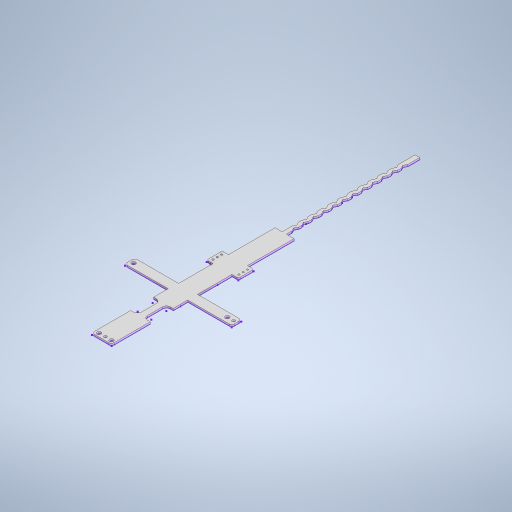
# Autodesk Inventor part: Thumb Finger Part
Saved by Autodesk Inventor 2023.1 (Build 271208000, 208)
## iProperties
Created: 2022-09-21
Part Number: Thumb Finger Part
Material: Generic
Document SubType Name: Modeling
Designer: lxpe222
Density: 1 g/cm^3
Appearance: Default
Author: lxpe222
Autodesk Inventor part; units mm, degrees
ref_plane "YZ Plane" through (0, 0, 0) normal (1, 0, 0) x (0, 1, 0)
ref_plane "XZ Plane" through (0, 0, 0) normal (0, 1, 0) x (-1, 0, 0)
ref_plane "XY Plane" through (0, 0, 0) normal (0, 0, 1) x (1, 0, 0)
sketch "Sketch1" plane through (0, 0, 0) normal (0, 1, 0) x (-1, 0, 0)
  line L0 (-8.7606, 60.7366) -> (-8.7606, 52.244)
  line L1 (2.2646, -7.3452) -> (2.2646, 17.544)
  line L2 (-8.811, 74.1038) -> (-8.811, 95.1313)
  line L3 (-7.311, 96.6313) -> (1.089, 96.6313)
  line L4 (2.589, 95.1313) -> (2.589, 74.061)
  circle A0 centre (0.414, 94.6613) radius 1.175
  circle A1 centre (-6.816, 94.6613) radius 1.175
  line L5 (-8.7606, 60.7366) -> (-7.0943, 60.7366)
  line L6 (-4.8143, 63.0166) -> (-4.8143, 71.8238)
  line L7 (-7.0943, 74.1038) -> (-8.811, 74.1038)
  line L8 (2.589, 74.061) -> (0.9294, 74.061)
  line L9 (-1.3506, 71.781) -> (-1.3506, 63.0166)
  line L10 (0.9294, 60.7366) -> (2.6222, 60.7366)
  arc A2 (0.9294, 74.061) -> (-1.3506, 71.781) centre (0.9294, 71.781) ccw
  arc A3 (-1.3506, 63.0166) -> (0.9294, 60.7366) centre (0.9294, 63.0166) ccw
  arc A4 (-7.0943, 60.7366) -> (-4.8143, 63.0166) centre (-7.0943, 63.0166) ccw
  arc A5 (-4.8143, 71.8238) -> (-7.0943, 74.1038) centre (-7.0943, 71.8238) ccw
  line L11 (2.6222, 52.244) -> (26.2646, 52.244)
  line L12 (27.7646, 50.744) -> (27.7646, 48.044)
  line L13 (26.2646, 46.544) -> (2.2646, 46.544)
  line L14 (-8.7606, 52.244) -> (-32.7606, 52.244)
  line L15 (-34.2606, 50.744) -> (-34.2606, 48.044)
  line L16 (-32.7606, 46.544) -> (-8.7606, 46.544)
  line L17 (2.2646, 26.544) -> (4.9546, 26.544)
  line L18 (5.9546, 25.544) -> (5.9546, 18.544)
  line L19 (4.9546, 17.544) -> (2.2646, 17.544)
  line L20 (-8.7606, 26.544) -> (-11.4506, 26.544)
  line L21 (-12.4506, 25.544) -> (-12.4506, 18.544)
  line L22 (-11.4506, 17.544) -> (-8.7606, 17.544)
  circle A6 centre (-3.2163, 94.6113) radius 0.85
  circle A7 centre (-28.8843, 49.394) radius 1.2
  circle A8 centre (-32.5093, 49.394) radius 0.825
  circle A9 centre (25.5896, 49.394) radius 1.2
  line L23 (2.6222, 52.244) -> (2.6222, 60.7366)
  line L24 (-8.7606, 17.544) -> (-8.7606, -9.5531)
  arc A10 (2.589, 95.1313) -> (1.089, 96.6313) centre (1.089, 95.1313) ccw
  arc A11 (-7.311, 96.6313) -> (-8.811, 95.1313) centre (-7.311, 95.1313) ccw
  arc A12 (26.2646, 46.544) -> (27.7646, 48.044) centre (26.2646, 48.044) ccw
  arc A13 (27.7646, 50.744) -> (26.2646, 52.244) centre (26.2646, 50.744) ccw
  arc A14 (-34.2606, 48.044) -> (-32.7606, 46.544) centre (-32.7606, 48.044) ccw
  arc A15 (-32.7606, 52.244) -> (-34.2606, 50.744) centre (-32.7606, 50.744) ccw
  line L25 (-4.2606, -9.5527) -> (-4.2468, -12.4286)
  line L26 (-1.8233, -14.9375) -> (-1.8491, -9.5528)
  line L27 (-8.7606, -9.5531) -> (-4.2606, -9.5528)
  line L28 (-4.2167, -68.4873) -> (-4.2167, -70.4904)
  line L29 (-2.7339, -69.436) -> (-1.6273, -67.5846)
  line L30 (-3.1633, -66.6169) -> (-4.2167, -68.4873)
  line L31 (-1.6273, -65.5835) -> (-1.6273, -67.5846)
  line L32 (-3.1633, -66.6169) -> (-4.2167, -64.7373)
  line L33 (-2.6377, -63.8108) -> (-1.6273, -65.5835)
  line L34 (-4.2167, -64.7373) -> (-4.2167, -62.7373)
  line L35 (-1.701, -26.8084) -> (-2.7095, -28.7084)
  line L36 (-4.2214, -28.1115) -> (-4.2214, -30.1115)
  line L37 (-2.7095, -28.7084) -> (-1.6807, -30.5584)
  line L38 (-1.6807, -32.5584) -> (-1.6807, -30.5584)
  line L39 (-3.1648, -32.0115) -> (-4.2214, -30.1115)
  line L40 (-1.6896, -38.3084) -> (-2.7534, -40.2084)
  line L41 (-2.7534, -40.2084) -> (-1.6666, -42.0584)
  line L42 (-3.1482, -43.5109) -> (-4.2333, -41.6115)
  line L43 (-1.6666, -44.0584) -> (-1.6666, -42.0584)
  line L44 (-1.6666, -44.0584) -> (-2.7357, -45.9584)
  line L45 (-4.299, -45.3609) -> (-3.1482, -43.5109)
  line L46 (-4.2333, -39.6115) -> (-4.2333, -41.6115)
  line L47 (-4.2333, -39.6115) -> (-3.1706, -37.7615)
  line L48 (-1.6896, -38.3084) -> (-1.6896, -36.3084)
  line L49 (-3.1706, -37.7615) -> (-4.2244, -35.8615)
  line L50 (-2.7156, -34.4584) -> (-1.6896, -36.3084)
  line L51 (-4.2244, -33.8615) -> (-4.2244, -35.8615)
  line L52 (-3.2118, -14.7615) -> (-0.6911, -14.7642) construction
  line L53 (-4.2824, -16.6115) -> (-3.2118, -14.7615)
  line L54 (-4.2824, -16.6115) -> (-4.2824, -18.6115)
  line L55 (-2.8081, -17.2084) -> (-1.731, -19.0584)
  line L56 (-3.2222, -20.5115) -> (-4.2824, -18.6115)
  line L57 (-1.731, -21.0584) -> (-1.731, -19.0584)
  line L58 (-3.2118, -14.7615) -> (-4.2468, -12.9643)
  line L59 (-4.2214, -28.1115) -> (-3.1802, -26.2615)
  line L60 (-1.701, -26.8084) -> (-1.701, -24.8084)
  line L61 (-3.1802, -26.2615) -> (-4.2412, -24.3615)
  line L62 (-2.7341, -22.9584) -> (-1.701, -24.8084)
  line L63 (-4.2412, -22.3615) -> (-4.2412, -24.3615)
  line L64 (-4.2412, -22.3615) -> (-3.2222, -20.5115)
  line L65 (-1.731, -21.0584) -> (-2.7341, -22.9584)
  line L66 (-3.1743, -49.2607) -> (-4.299, -47.3609)
  line L67 (-4.3381, -51.1107) -> (-3.1743, -49.2607)
  line L68 (-2.6912, -52.2338) -> (-1.5867, -54.0838)
  line L69 (-4.3381, -51.1107) -> (-4.3381, -53.1107)
  line L70 (-1.7329, -50.3338) -> (-2.6912, -52.2338)
  line L71 (-1.7329, -50.3338) -> (-1.6601, -49.8084)
  line L72 (-1.6601, -49.8084) -> (-1.6601, -47.8084)
  line L73 (-2.7357, -45.9584) -> (-1.6601, -47.8084)
  line L74 (-4.299, -45.3609) -> (-4.299, -47.3609)
  line L75 (-1.6807, -32.5584) -> (-2.7156, -34.4584)
  line L76 (-4.2244, -33.8615) -> (-3.1648, -32.0115)
  line L77 (-2.7339, -69.436) -> (-1.7343, -71.333)
  line L78 (-3.2659, -72.3279) -> (-4.2167, -70.4904)
  line L79 (-1.7343, -71.333) -> (-1.7343, -73.333)
  line L80 (-3.2659, -72.3279) -> (-4.425, -74.2346)
  line L81 (-2.7876, -75.2268) -> (-1.7343, -73.333)
  line L82 (-2.7876, -75.2268) -> (-1.7343, -77.083)
  line L83 (-4.425, -74.2346) -> (-4.425, -76.2346)
  line L84 (-3.2287, -55.1137) -> (-4.3381, -53.1107)
  line L85 (-1.5867, -54.0838) -> (-1.5867, -56.0838)
  line L86 (-3.2287, -55.1137) -> (-4.3098, -56.9885)
  line L87 (-2.6396, -58.004) -> (-1.5867, -56.0838)
  line L88 (-4.3098, -56.9885) -> (-4.313, -58.9885)
  line L89 (-2.6396, -58.004) -> (-1.5867, -59.8338)
  line L90 (-3.2112, -60.8694) -> (-4.313, -58.9885)
  line L91 (-3.2112, -60.8694) -> (-4.2167, -62.7373)
  line L92 (-2.6377, -63.8108) -> (-1.5867, -61.8338)
  line L93 (-1.5867, -59.8338) -> (-1.5867, -61.8338)
  line L94 (-3.372, -78.0699) -> (-4.425, -79.9846)
  line L95 (-3.372, -78.0699) -> (-4.425, -76.2346)
  line L96 (-4.425, -86.9746) -> (-4.425, -79.9846)
  line L97 (-1.7343, -86.9746) -> (-4.425, -86.9746)
  line L98 (-1.7343, -77.083) -> (-1.7343, -86.9746)
  line L99 (-1.8233, -14.9375) -> (-1.8233, -15.4921)
  line L100 (-1.8233, -15.4921) -> (-2.8081, -17.2084)
  line L101 (-4.2468, -12.4286) -> (-4.2468, -12.9643)
  line L102 (-1.8491, -9.5528) -> (2.2646, -9.5528)
  line L103 (2.2646, -9.5528) -> (2.2646, -7.3452)
  line L104 (2.2646, 26.544) -> (2.2646, 46.544)
  line L105 (-8.7606, 26.544) -> (-8.7606, 46.544)
  circle A16 centre (4.2946, 22.044) radius 0.5
  circle A17 centre (4.2946, 19.544) radius 0.5
  circle A18 centre (4.2946, 24.544) radius 0.5
  circle A19 centre (-10.7906, 22.044) radius 0.5
  circle A20 centre (-10.7906, 19.544) radius 0.5
  circle A21 centre (-10.7906, 24.544) radius 0.5
  arc A22 (4.9546, 17.544) -> (5.9546, 18.544) centre (4.9546, 18.544) ccw
  arc A23 (5.9546, 25.544) -> (4.9546, 26.544) centre (4.9546, 25.544) ccw
  arc A24 (-11.4506, 26.544) -> (-12.4506, 25.544) centre (-11.4506, 25.544) ccw
  arc A25 (-12.4506, 18.544) -> (-11.4506, 17.544) centre (-11.4506, 18.544) ccw
  point P0 (-8.811, 96.6313)
  point P1 (2.589, 96.6313)
  point P2 (-6.9279, 18.3671)
  point P3 (0.6606, 18.3671)
  point P4 (-6.9323, 25.0551)
  point P5 (27.7646, 46.544)
  point P6 (27.7646, 52.244)
  point P7 (-34.2606, 46.544)
  point P8 (-34.2606, 52.244)
  point P9 (2.2646, 46.9721)
  point P10 (-8.7606, 35.0882)
  point P11 (5.9546, 17.544)
  point P12 (5.9546, 26.544)
  point P13 (-12.4506, 17.544)
  point P14 (-12.4506, 26.544)
  point P15 (-3.6908, -42.5612)
  point P16 (-3.7523, -19.5615)
  point P17 (-3.7317, -21.4365)
  point P18 (-3.7367, -48.3108)
  point P19 (-2.139, -53.1588)
  point P20 (2.6394, 52.7)
  point P21 (-8.7606, 56.4903)
  point P22 (3.6096, 26.544)
  dimension "d276" = 2.4
  dimension "d277" = 2.4
  dimension "d280" = 1.5
  dimension "d281" = 2.35
  dimension "d282" = 2.35
  dimension "d284" = 1.65
  dimension "d286" = 1.7
  dimension "d288" = 0.795
  dimension "d289" = 0.795
  dimension "d290" = 1.17
  dimension "d291" = 1.6
  dimension "d292" = 1.575
  dimension "d293" = 1.5
  dimension "d294" = 1.5
  dimension "d296" = 0.975
  dimension "d297" = 2.175
  dimension "d312" = 0.9263
  dimension "d313" = 120
  dimension "d315" = 2
  dimension "d316" = 2
  dimension "d317" = 2
  dimension "d318" = 2
  dimension "d319" = 2
  dimension "d320" = 2
  dimension "d321" = 2
  dimension "d322" = 2
  dimension "d323" = 2
  dimension "d324" = 2
  dimension "d325" = 2
  dimension "d326" = 2
  dimension "d327" = 2
  dimension "d328" = 2
  dimension "d329" = 2
  dimension "d330" = 2.0032
  dimension "d331" = 2
  dimension "d332" = 2
  dimension "d333" = 3.75
  dimension "d334" = 3.75
  dimension "d335" = 3.75
  dimension "d336" = 3.75
  dimension "d337" = 3.75
  dimension "d338" = 3.75
  dimension "d339" = 3.75
  dimension "d340" = 3.75
  dimension "d341" = 3.75
  dimension "d342" = 3.75
  dimension "d343" = 3.75
  dimension "d344" = 3.75
  dimension "d347" = 1.85
  dimension "d348" = 1.85
  dimension "d349" = 1.85
  dimension "d350" = 1.85
  dimension "d351" = 1.85
  dimension "d352" = 1.85
  dimension "d353" = 1.85
  dimension "d354" = 1.85
  dimension "d355" = 1.85
  dimension "d356" = 1.85
  dimension "d357" = 1.85
  dimension "d358" = 1.85
  dimension "d359" = 1.85
  dimension "d360" = 1.85
  dimension "d361" = 3.75
  dimension "d362" = 121.346
  constraints: 213 end point, 58 parallel, 28 point on circle, 28 point on line, 28 tangent, 26 centre point, 9 equal radius, 9 perpendicular, 9 vertical, 7 horizontal, 7 midpoint, 1 collinear
  measures "d276" diameter of A7
  measures "d277" diameter of A9
  measures "d280" radius of A10
  measures "d281" diameter of A0
  measures "d282" diameter of A1
  measures "d284" diameter of A8
  measures "d286" diameter of A6
  measures "d288" distance edge to line of A1 L3
  measures "d289" distance edge to line of A0 L3
  measures "d290" distance edge to line of A6 L3
  measures "d293" radius of A12
  measures "d294" radius of A14
  measures "d296" distance edge to line of A9 L12
  measures "d297" distance from line of L4 A0.centre
  measures "d312" distance edge to line of A8 L15
  measures "d313" angle of L52 L58
  measures "d315" distance of L57.start L55.end
  measures "d316" distance of L53.start L56.end
  measures "d317" distance of L63.start L61.end
  measures "d318" distance of L35.start L60.end
  measures "d319" distance of L59.start L39.end
  measures "d320" distance of L75.start L38.end
  measures "d321" distance of L51.start L49.end
  measures "d322" distance of L40.start L48.end
  measures "d323" distance of L47.start L46.end
  measures "d324" distance of L44.start L41.end
  measures "d325" distance of L74.start L66.end
  measures "d326" distance of L71.end L72.end
  measures "d327" distance of L67.start L69.end
  measures "d328" distance from line of point (-3.752, -19.561) L55
  measures "d329" distance between parallel lines of L61 L62
  measures "d330" distance between parallel lines of L39 L37
  measures "d331" distance between parallel lines of L49 L50
  measures "d332" distance from line of point (-3.691, -42.561) L41
  measures "d333" vertical distance of L85.start L71.start
  measures "d334" distance of L66.end L67.start
  measures "d335" distance of L72.end L44.start
  measures "d336" vertical distance of L40.start L41.end
  measures "d337" distance of L74.start L46.end
  measures "d338" distance of L49.end L47.start
  measures "d339" distance of L75.start L48.end
  measures "d340" distance of L39.end L51.start
  measures "d341" vertical distance of L61.end L59.start
  measures "d342" vertical distance of L35.start L38.end
  measures "d343" vertical distance of L57.start L60.end
  measures "d344" vertical distance of L56.end L63.start
  measures "d347" vertical distance of L53.start L58.start
  measures "d348" vertical distance of L63.start L56.start
  measures "d349" vertical distance of L55.start L55.end
  measures "d350" vertical distance of L62.start L60.end
  measures "d351" vertical distance of L59.start L59.end
  measures "d352" vertical distance of L38.end L35.end
  measures "d353" vertical distance of L51.start L76.end
  measures "d354" vertical distance of L50.start L48.end
  measures "d355" vertical distance of L49.start L47.start
  measures "d356" vertical distance of L40.end L41.end
  measures "d357" vertical distance of L73.start L72.end
  measures "d358" vertical distance of L45.end L74.start
  measures "d359" vertical distance of L67.start L67.end
  measures "d360" vertical distance of L70.end L85.start
  measures "d361" distance of L83.end L94.end
  measures "d362" angle of L94 L95
extrude "Extrusion8" add sketch "Sketch1" along normal blind 1
body "Solid3"
